Autodesk Inventor part; units mm, degrees
(part 3 of 3)
  spline S74 degree 3 poles (635.3276, -322.5137) (634.4201, -321.4591) (632.6051, -319.35) (629.8185, -316.2423) (626.9841, -313.1784) (624.099, -310.1618) (621.1497, -307.2086) (618.9244, -305.0061) (617.3793, -303.6029) (616.7979, -302.9531) (616.3991, -302.3815) (616.1608, -301.9167) (615.9496, -301.4385) (615.8138, -300.9335) (615.7143, -300.4207) (615.6711, -299.7252) (615.7494, -299.0281) (615.9357, -298.3567) (616.2141, -297.7178) (616.6068, -296.9422) (616.9684, -296.1515) (617.2943, -295.5356) (617.703, -294.9713) (618.1993, -294.4755) (618.77, -294.0756) (619.2329, -293.8336) (619.7124, -293.625) (620.2179, -293.4919) (620.73, -293.3884) (621.4255, -293.3439) (622.296, -293.3933) (624.3564, -293.7264) (627.4658, -294.093) (631.6136, -294.5575) (635.7709, -294.9324) (639.9336, -295.2381) (644.1007, -295.4791) (646.8813, -295.5831) (648.2716, -295.6351) knots 0 0 0 0 0.062506 0.125011 0.187517 0.250023 0.312528 0.375034 0.390661 0.406272 0.414085 0.421898 0.429707 0.43752 0.44533 0.453144 0.468748 0.476562 0.484374 0.5 0.515626 0.523438 0.531252 0.546856 0.55467 0.56248 0.570293 0.578102 0.585915 0.593728 0.609339 0.624966 0.687472 0.749977 0.812483 0.874989 0.937494 1 1 1 1 projected
  arc A78 (648.2716, -295.6351) -> (652.4116, -286.3832) centre (0, 0) ccw projected
  spline S75 degree 3 poles (652.4116, -286.3832) (651.4464, -285.3812) (649.5159, -283.3772) (646.5595, -280.4306) (643.5578, -277.5304) (640.508, -274.6804) (637.3978, -271.8971) (635.0525, -269.8229) (633.4312, -268.5085) (632.8143, -267.8923) (632.3841, -267.3441) (632.12, -266.8933) (631.8824, -266.4277) (631.7185, -265.9312) (631.5904, -265.4247) (631.5083, -264.7327) (631.5473, -264.0323) (631.6957, -263.3515) (631.9378, -262.6981) (632.2864, -261.9016) (632.6031, -261.0919) (632.894, -260.4587) (633.2704, -259.8724) (633.7381, -259.3495) (634.2855, -258.9182) (634.7342, -258.6507) (635.2012, -258.4155) (635.6984, -258.2543) (636.2039, -258.1223) (636.8958, -258.0388) (637.7677, -258.0393) (639.8435, -258.2563) (642.9686, -258.448) (647.1359, -258.6792) (651.3077, -258.8204) (655.481, -258.8923) (659.655, -258.8992) (662.4371, -258.8472) (663.8282, -258.8212) knots 0 0 0 0 0.062506 0.125011 0.187517 0.250023 0.312528 0.375034 0.390661 0.406272 0.414085 0.421898 0.429707 0.43752 0.44533 0.453144 0.468748 0.476562 0.484374 0.5 0.515626 0.523438 0.531252 0.546856 0.55467 0.56248 0.570293 0.578102 0.585915 0.593728 0.609339 0.624966 0.687472 0.749977 0.812483 0.874989 0.937494 1 1 1 1 projected
  arc A79 (663.8282, -258.8212) -> (667.4429, -249.3517) centre (0, 0) ccw projected
  spline S76 degree 3 poles (667.4429, -249.3517) (666.423, -248.4053) (664.3832, -246.5127) (661.2662, -243.7365) (658.1066, -241.0092) (654.9019, -238.3347) (651.6405, -235.7302) (649.1825, -233.7907) (647.4901, -232.5693) (646.8396, -231.9887) (646.3793, -231.4654) (646.0904, -231.0302) (645.8271, -230.5786) (645.6356, -230.0921) (645.4793, -229.5936) (645.3585, -228.9073) (645.3582, -228.2058) (645.4682, -227.5178) (645.6733, -226.8518) (645.9767, -226.037) (646.2475, -225.2109) (646.5024, -224.5623) (646.8453, -223.9558) (647.2829, -223.4075) (647.8053, -222.9463) (648.2383, -222.654) (648.6914, -222.393) (649.1788, -222.2041) (649.676, -222.044) (650.3622, -221.9218) (651.2327, -221.8734) (653.3175, -221.9737) (656.4484, -221.9899) (660.6221, -221.9871) (664.7953, -221.8941) (668.966, -221.7319) (673.1339, -221.5048) (675.9087, -221.2968) (677.2961, -221.1928) knots 0 0 0 0 0.062506 0.125011 0.187517 0.250023 0.312528 0.375034 0.390661 0.406272 0.414085 0.421898 0.429707 0.43752 0.44533 0.453144 0.468748 0.476562 0.484374 0.5 0.515626 0.523438 0.531252 0.546856 0.55467 0.56248 0.570293 0.578102 0.585915 0.593728 0.609339 0.624966 0.687472 0.749977 0.812483 0.874989 0.937494 1 1 1 1 projected
  arc A80 (677.2961, -221.1928) -> (680.3741, -211.5356) centre (0, 0) ccw projected
  spline S77 degree 3 poles (680.3741, -211.5356) (679.3028, -210.6479) (677.1601, -208.8726) (673.8923, -206.2756) (670.5848, -203.7298) (667.2351, -201.2391) (663.8328, -198.8216) (661.27, -197.023) (659.5117, -195.8984) (658.8297, -195.3552) (658.3408, -194.8585) (658.028, -194.4401) (657.7397, -194.0041) (657.5212, -193.529) (657.3372, -193.0401) (657.1782, -192.3616) (657.1385, -191.6613) (657.2098, -190.9681) (657.3772, -190.2917) (657.6344, -189.4612) (657.8585, -188.6212) (658.0766, -187.9593) (658.385, -187.3345) (658.7912, -186.7626) (659.2869, -186.2728) (659.7028, -185.9567) (660.1405, -185.6707) (660.6166, -185.4548) (661.1041, -185.267) (661.7823, -185.1066) (662.6487, -185.0095) (664.7358, -184.9927) (667.8628, -184.8333) (672.0298, -184.5965) (676.1911, -184.2697) (680.3462, -183.8738) (684.4948, -183.4134) (687.2536, -183.0502) (688.6329, -182.8686) knots 0 0 0 0 0.062506 0.125011 0.187517 0.250023 0.312528 0.375034 0.390661 0.406272 0.414085 0.421898 0.429707 0.43752 0.44533 0.453144 0.468748 0.476562 0.484374 0.5 0.515626 0.523438 0.531252 0.546856 0.55467 0.56248 0.570293 0.578102 0.585915 0.593728 0.609339 0.624966 0.687472 0.749977 0.812483 0.874989 0.937494 1 1 1 1 projected
  arc A81 (688.6329, -182.8686) -> (691.1647, -173.0539) centre (0, 0) ccw projected
  spline S78 degree 3 poles (691.1647, -173.0539) (690.0452, -172.2277) (687.8064, -170.5754) (684.3981, -168.1656) (680.953, -165.8093) (677.469, -163.5103) (673.9365, -161.2874) (671.2769, -159.6353) (669.4583, -158.6111) (668.7469, -158.1069) (668.2309, -157.6385) (667.8951, -157.2383) (667.5829, -156.8191) (667.3381, -156.357) (667.127, -155.8792) (666.9301, -155.2107) (666.8512, -154.5137) (666.8835, -153.8177) (667.0128, -153.1329) (667.223, -152.2893) (667.3996, -151.438) (667.5803, -150.765) (667.8532, -150.1239) (668.2267, -149.5301) (668.6941, -149.0132) (669.0916, -148.6743) (669.5126, -148.3642) (669.9759, -148.122) (670.452, -147.9072) (671.1202, -147.709) (671.9798, -147.5634) (674.0627, -147.4297) (677.1758, -147.0952) (681.3229, -146.6251) (685.4594, -146.0655) (689.5858, -145.4372) (693.702, -144.7449) (696.4361, -144.2276) (697.8031, -143.9689) knots 0 0 0 0 0.062506 0.125011 0.187517 0.250023 0.312528 0.375034 0.390661 0.406272 0.414085 0.421898 0.429707 0.43752 0.44533 0.453144 0.468748 0.476562 0.484374 0.5 0.515626 0.523438 0.531252 0.546856 0.55467 0.56248 0.570293 0.578102 0.585915 0.593728 0.609339 0.624966 0.687472 0.749977 0.812483 0.874989 0.937494 1 1 1 1 projected
  arc A82 (697.8031, -143.9689) -> (699.7805, -134.0277) centre (0, 0) ccw projected
  spline S79 degree 3 poles (699.7805, -134.0277) (698.6166, -133.2656) (696.2886, -131.7414) (692.7506, -129.5266) (689.1788, -127.3671) (685.5713, -125.2671) (681.9197, -123.2458) (679.1716, -121.7454) (677.2985, -120.8247) (676.56, -120.3613) (676.0185, -119.9225) (675.6608, -119.5418) (675.3255, -119.1407) (675.0552, -118.6931) (674.8177, -118.2279) (674.5836, -117.5715) (674.4658, -116.88) (674.459, -116.1832) (674.5497, -115.4923) (674.7123, -114.6382) (674.8409, -113.7784) (674.9835, -113.0963) (675.22, -112.4409) (675.5596, -111.8271) (675.9973, -111.2848) (676.3752, -110.9241) (676.7782, -110.5909) (677.2271, -110.3231) (677.6905, -110.0819) (678.3465, -109.8466) (679.1966, -109.6531) (681.2687, -109.4027) (684.3582, -108.8942) (688.4724, -108.1923) (692.571, -107.4016) (696.6556, -106.5431) (700.7266, -105.621) (703.4274, -104.9512) (704.7778, -104.6163) knots 0 0 0 0 0.062506 0.125011 0.187517 0.250023 0.312528 0.375034 0.390661 0.406272 0.414085 0.421898 0.429707 0.43752 0.44533 0.453144 0.468748 0.476562 0.484374 0.5 0.515626 0.523438 0.531252 0.546856 0.55467 0.56248 0.570293 0.578102 0.585915 0.593728 0.609339 0.624966 0.687472 0.749977 0.812483 0.874989 0.937494 1 1 1 1 projected
  arc A83 (704.7778, -104.6163) -> (706.1947, -94.5799) centre (0, 0) ccw projected
  spline S80 degree 3 poles (706.1947, -94.5799) (704.9898, -93.8842) (702.58, -92.4929) (698.9234, -90.48) (695.2361, -88.5241) (691.5166, -86.6297) (687.7574, -84.8163) (684.9295, -83.4724) (683.0077, -82.6582) (682.2443, -82.2369) (681.6791, -81.8292) (681.3006, -81.4691) (680.9434, -81.0875) (680.6484, -80.6558) (680.3852, -80.2045) (680.1147, -79.5623) (679.9583, -78.8785) (679.9124, -78.1832) (679.9642, -77.4883) (680.0787, -76.6265) (680.1588, -75.7608) (680.263, -75.0717) (680.4624, -74.4041) (680.7671, -73.7722) (681.1737, -73.2063) (681.5307, -72.825) (681.9144, -72.4697) (682.3476, -72.1771) (682.7967, -71.9103) (683.4385, -71.6386) (684.2764, -71.3977) (686.3312, -71.0316) (689.3873, -70.3506) (693.4557, -69.4192) (697.5035, -68.3999) (701.5336, -67.3136) (705.5465, -66.1648) (708.2054, -65.3446) (709.5349, -64.9345) knots 0 0 0 0 0.062506 0.125011 0.187517 0.250023 0.312528 0.375034 0.390661 0.406272 0.414085 0.421898 0.429707 0.43752 0.44533 0.453144 0.468748 0.476562 0.484374 0.5 0.515626 0.523438 0.531252 0.546856 0.55467 0.56248 0.570293 0.578102 0.585915 0.593728 0.609339 0.624966 0.687472 0.749977 0.812483 0.874989 0.937494 1 1 1 1 projected
  arc A84 (709.5349, -64.9345) -> (710.3868, -54.8344) centre (0, 0) ccw projected
  spline S81 degree 3 poles (710.3868, -54.8344) (709.1448, -54.2075) (706.6608, -52.9535) (702.8971, -51.1487) (699.1059, -49.4027) (695.286, -47.7198) (691.4311, -46.12) (688.5323, -44.9368) (686.5679, -44.2317) (685.7821, -43.8538) (685.1949, -43.4784) (684.7968, -43.1401) (684.4188, -42.7791) (684.1, -42.3646) (683.8119, -41.9289) (683.5058, -41.3028) (683.3113, -40.6288) (683.2266, -39.9372) (683.2393, -39.2405) (683.3053, -38.3736) (683.3367, -37.5048) (683.4021, -36.811) (683.5638, -36.1332) (683.8325, -35.4853) (684.2068, -34.8974) (684.5419, -34.4967) (684.905, -34.1205) (685.3211, -33.8041) (685.7546, -33.5125) (686.3801, -33.2052) (687.2032, -32.9177) (689.2343, -32.4369) (692.2473, -31.5857) (696.2572, -30.4276) (700.2414, -29.183) (704.2043, -27.8724) (708.1464, -26.5004) (710.7552, -25.5324) (712.0596, -25.0484) knots 0 0 0 0 0.062506 0.125011 0.187517 0.250023 0.312528 0.375034 0.390661 0.406272 0.414085 0.421898 0.429707 0.43752 0.44533 0.453144 0.468748 0.476562 0.484374 0.5 0.515626 0.523438 0.531252 0.546856 0.55467 0.56248 0.570293 0.578102 0.585915 0.593728 0.609339 0.624966 0.687472 0.749977 0.812483 0.874989 0.937494 1 1 1 1 projected
  arc A85 (712.0596, -25.0484) -> (712.3438, -14.9165) centre (0, 0) ccw projected
  spline S82 degree 3 poles (712.3438, -14.9165) (711.0686, -14.3601) (708.5182, -13.2474) (704.6592, -11.6564) (700.7761, -10.1258) (696.8679, -8.6597) (692.9293, -7.2786) (689.9687, -6.2598) (687.9678, -5.6659) (687.1621, -5.3327) (686.5548, -4.9908) (686.1384, -4.6754) (685.7407, -4.3362) (685.3992, -3.9402) (685.0871, -3.5213) (684.7464, -2.9134) (684.5144, -2.2513) (684.391, -1.5656) (684.3646, -0.8692) (684.3819, 0) (684.3646, 0.8692) (684.391, 1.5656) (684.5144, 2.2513) (684.7464, 2.9134) (685.0871, 3.5213) (685.3992, 3.9402) (685.7407, 4.3362) (686.1384, 4.6754) (686.5548, 4.9908) (687.1621, 5.3327) (687.9678, 5.6659) (689.9687, 6.2598) (692.9293, 7.2786) (696.8679, 8.6597) (700.7761, 10.1258) (704.6592, 11.6564) (708.5182, 13.2474) (711.0686, 14.3601) (712.3438, 14.9165) knots 0 0 0 0 0.062506 0.125011 0.187517 0.250023 0.312528 0.375034 0.390661 0.406272 0.414085 0.421898 0.429707 0.43752 0.44533 0.453144 0.468748 0.476562 0.484374 0.5 0.515626 0.523438 0.531252 0.546856 0.55467 0.56248 0.570293 0.578102 0.585915 0.593728 0.609339 0.624966 0.687472 0.749977 0.812483 0.874989 0.937494 1 1 1 1 projected
  arc A86 (712.3438, 14.9165) -> (712.0596, 25.0484) centre (0, 0) ccw projected
  spline S83 degree 3 poles (712.0596, 25.0484) (710.7552, 25.5324) (708.1464, 26.5004) (704.2043, 27.8724) (700.2414, 29.183) (696.2572, 30.4276) (692.2473, 31.5857) (689.2343, 32.4369) (687.2032, 32.9177) (686.3801, 33.2052) (685.7546, 33.5125) (685.3211, 33.8041) (684.905, 34.1205) (684.5419, 34.4967) (684.2068, 34.8974) (683.8325, 35.4853) (683.5638, 36.1332) (683.4021, 36.811) (683.3367, 37.5048) (683.3053, 38.3736) (683.2393, 39.2405) (683.2266, 39.9372) (683.3113, 40.6288) (683.5058, 41.3028) (683.8119, 41.9289) (684.1, 42.3646) (684.4188, 42.7791) (684.7968, 43.1401) (685.1949, 43.4784) (685.7821, 43.8538) (686.5679, 44.2317) (688.5323, 44.9368) (691.4311, 46.12) (695.286, 47.7198) (699.1059, 49.4027) (702.8971, 51.1487) (706.6608, 52.9535) (709.1448, 54.2075) (710.3868, 54.8344) knots 0 0 0 0 0.062506 0.125011 0.187517 0.250023 0.312528 0.375034 0.390661 0.406272 0.414085 0.421898 0.429707 0.43752 0.44533 0.453144 0.468748 0.476562 0.484374 0.5 0.515626 0.523438 0.531252 0.546856 0.55467 0.56248 0.570293 0.578102 0.585915 0.593728 0.609339 0.624966 0.687472 0.749977 0.812483 0.874989 0.937494 1 1 1 1 projected
  arc A87 (710.3868, 54.8344) -> (709.5349, 64.9345) centre (0, 0) ccw projected
  spline S84 degree 3 poles (709.5349, 64.9345) (708.2054, 65.3446) (705.5465, 66.1648) (701.5336, 67.3136) (697.5035, 68.3999) (693.4557, 69.4192) (689.3873, 70.3506) (686.3312, 71.0316) (684.2764, 71.3977) (683.4385, 71.6386) (682.7967, 71.9103) (682.3476, 72.1771) (681.9144, 72.4697) (681.5307, 72.825) (681.1737, 73.2063) (680.7671, 73.7722) (680.4624, 74.4041) (680.263, 75.0717) (680.1588, 75.7608) (680.0787, 76.6265) (679.9642, 77.4883) (679.9124, 78.1832) (679.9583, 78.8785) (680.1147, 79.5623) (680.3852, 80.2045) (680.6484, 80.6558) (680.9434, 81.0875) (681.3006, 81.4691) (681.6791, 81.8292) (682.2443, 82.2369) (683.0077, 82.6582) (684.9295, 83.4724) (687.7574, 84.8163) (691.5166, 86.6297) (695.2361, 88.5241) (698.9234, 90.48) (702.58, 92.4929) (704.9898, 93.8842) (706.1947, 94.5799) knots 0 0 0 0 0.062506 0.125011 0.187517 0.250023 0.312528 0.375034 0.390661 0.406272 0.414085 0.421898 0.429707 0.43752 0.44533 0.453144 0.468748 0.476562 0.484374 0.5 0.515626 0.523438 0.531252 0.546856 0.55467 0.56248 0.570293 0.578102 0.585915 0.593728 0.609339 0.624966 0.687472 0.749977 0.812483 0.874989 0.937494 1 1 1 1 projected
  arc A88 (706.1947, 94.5799) -> (704.7778, 104.6163) centre (0, 0) ccw projected
  spline S85 degree 3 poles (704.7778, 104.6163) (703.4274, 104.9512) (700.7266, 105.621) (696.6556, 106.5431) (692.571, 107.4016) (688.4724, 108.1923) (684.3582, 108.8942) (681.2687, 109.4027) (679.1966, 109.6531) (678.3465, 109.8466) (677.6905, 110.0819) (677.2271, 110.3231) (676.7782, 110.5909) (676.3752, 110.9241) (675.9973, 111.2848) (675.5596, 111.8271) (675.22, 112.4409) (674.9835, 113.0963) (674.8409, 113.7784) (674.7123, 114.6382) (674.5497, 115.4923) (674.459, 116.1832) (674.4658, 116.88) (674.5836, 117.5715) (674.8177, 118.2279) (675.0552, 118.6931) (675.3255, 119.1407) (675.6608, 119.5418) (676.0185, 119.9225) (676.56, 120.3613) (677.2985, 120.8247) (679.1716, 121.7454) (681.9197, 123.2458) (685.5713, 125.2671) (689.1788, 127.3671) (692.7506, 129.5266) (696.2886, 131.7414) (698.6166, 133.2656) (699.7805, 134.0277) knots 0 0 0 0 0.062506 0.125011 0.187517 0.250023 0.312528 0.375034 0.390661 0.406272 0.414085 0.421898 0.429707 0.43752 0.44533 0.453144 0.468748 0.476562 0.484374 0.5 0.515626 0.523438 0.531252 0.546856 0.55467 0.56248 0.570293 0.578102 0.585915 0.593728 0.609339 0.624966 0.687472 0.749977 0.812483 0.874989 0.937494 1 1 1 1 projected
  arc A89 (699.7805, 134.0277) -> (697.8031, 143.9689) centre (0, 0) ccw projected
  spline S86 degree 3 poles (697.8031, 143.9689) (696.4361, 144.2276) (693.702, 144.7449) (689.5858, 145.4372) (685.4594, 146.0655) (681.3229, 146.6251) (677.1758, 147.0952) (674.0627, 147.4297) (671.9798, 147.5634) (671.1202, 147.709) (670.452, 147.9072) (669.9759, 148.122) (669.5126, 148.3642) (669.0916, 148.6743) (668.6941, 149.0132) (668.2267, 149.5301) (667.8532, 150.1239) (667.5803, 150.765) (667.3996, 151.438) (667.223, 152.2893) (667.0128, 153.1329) (666.8835, 153.8177) (666.8512, 154.5137) (666.9301, 155.2107) (667.127, 155.8792) (667.3381, 156.357) (667.5829, 156.8191) (667.8951, 157.2383) (668.2309, 157.6385) (668.7469, 158.1069) (669.4583, 158.6111) (671.2769, 159.6353) (673.9365, 161.2874) (677.469, 163.5103) (680.953, 165.8093) (684.3981, 168.1656) (687.8064, 170.5754) (690.0452, 172.2277) (691.1647, 173.0539) knots 0 0 0 0 0.062506 0.125011 0.187517 0.250023 0.312528 0.375034 0.390661 0.406272 0.414085 0.421898 0.429707 0.43752 0.44533 0.453144 0.468748 0.476562 0.484374 0.5 0.515626 0.523438 0.531252 0.546856 0.55467 0.56248 0.570293 0.578102 0.585915 0.593728 0.609339 0.624966 0.687472 0.749977 0.812483 0.874989 0.937494 1 1 1 1 projected
  arc A90 (691.1647, 173.0539) -> (688.6329, 182.8686) centre (0, 0) ccw projected
  spline S87 degree 3 poles (688.6329, 182.8686) (687.2536, 183.0502) (684.4948, 183.4134) (680.3462, 183.8738) (676.1911, 184.2697) (672.0298, 184.5965) (667.8628, 184.8333) (664.7358, 184.9927) (662.6487, 185.0095) (661.7823, 185.1066) (661.1041, 185.267) (660.6166, 185.4548) (660.1405, 185.6707) (659.7028, 185.9567) (659.2869, 186.2728) (658.7912, 186.7626) (658.385, 187.3345) (658.0766, 187.9593) (657.8585, 188.6212) (657.6344, 189.4612) (657.3772, 190.2917) (657.2098, 190.9681) (657.1385, 191.6613) (657.1782, 192.3616) (657.3372, 193.0401) (657.5212, 193.529) (657.7397, 194.0041) (658.028, 194.4401) (658.3408, 194.8585) (658.8297, 195.3552) (659.5117, 195.8984) (661.27, 197.023) (663.8328, 198.8216) (667.2351, 201.2391) (670.5848, 203.7298) (673.8923, 206.2756) (677.1601, 208.8726) (679.3028, 210.6479) (680.3741, 211.5356) knots 0 0 0 0 0.062506 0.125011 0.187517 0.250023 0.312528 0.375034 0.390661 0.406272 0.414085 0.421898 0.429707 0.43752 0.44533 0.453144 0.468748 0.476562 0.484374 0.5 0.515626 0.523438 0.531252 0.546856 0.55467 0.56248 0.570293 0.578102 0.585915 0.593728 0.609339 0.624966 0.687472 0.749977 0.812483 0.874989 0.937494 1 1 1 1 projected
  arc A91 (680.3741, 211.5356) -> (677.2961, 221.1928) centre (0, 0) ccw projected
  spline S88 degree 3 poles (677.2961, 221.1928) (675.9087, 221.2968) (673.1339, 221.5048) (668.966, 221.7319) (664.7953, 221.8941) (660.6221, 221.9871) (656.4484, 221.9899) (653.3175, 221.9737) (651.2327, 221.8734) (650.3622, 221.9218) (649.676, 222.044) (649.1788, 222.2041) (648.6914, 222.393) (648.2383, 222.654) (647.8053, 222.9463) (647.2829, 223.4075) (646.8453, 223.9558) (646.5024, 224.5623) (646.2475, 225.2109) (645.9767, 226.037) (645.6733, 226.8518) (645.4682, 227.5178) (645.3582, 228.2058) (645.3585, 228.9073) (645.4793, 229.5936) (645.6356, 230.0921) (645.8271, 230.5786) (646.0904, 231.0302) (646.3793, 231.4654) (646.8396, 231.9887) (647.4901, 232.5693) (649.1825, 233.7907) (651.6405, 235.7302) (654.9019, 238.3347) (658.1066, 241.0092) (661.2662, 243.7365) (664.3832, 246.5127) (666.423, 248.4053) (667.4429, 249.3517) knots 0 0 0 0 0.062506 0.125011 0.187517 0.250023 0.312528 0.375034 0.390661 0.406272 0.414085 0.421898 0.429707 0.43752 0.44533 0.453144 0.468748 0.476562 0.484374 0.5 0.515626 0.523438 0.531252 0.546856 0.55467 0.56248 0.570293 0.578102 0.585915 0.593728 0.609339 0.624966 0.687472 0.749977 0.812483 0.874989 0.937494 1 1 1 1 projected
  arc A92 (667.4429, 249.3517) -> (663.8282, 258.8212) centre (0, 0) ccw projected
  spline S89 degree 3 poles (663.8282, 258.8212) (662.4371, 258.8472) (659.655, 258.8992) (655.481, 258.8923) (651.3077, 258.8204) (647.1359, 258.6792) (642.9686, 258.448) (639.8435, 258.2563) (637.7677, 258.0393) (636.8958, 258.0388) (636.2039, 258.1223) (635.6984, 258.2543) (635.2012, 258.4155) (634.7342, 258.6507) (634.2855, 258.9182) (633.7381, 259.3495) (633.2704, 259.8724) (632.894, 260.4587) (632.6031, 261.0919) (632.2864, 261.9016) (631.9378, 262.6981) (631.6957, 263.3515) (631.5473, 264.0323) (631.5083, 264.7327) (631.5904, 265.4247) (631.7185, 265.9312) (631.8824, 266.4277) (632.12, 266.8933) (632.3841, 267.3441) (632.8143, 267.8923) (633.4312, 268.5085) (635.0525, 269.8229) (637.3978, 271.8971) (640.508, 274.6804) (643.5578, 277.5304) (646.5595, 280.4306) (649.5159, 283.3772) (651.4464, 285.3812) (652.4116, 286.3832) knots 0 0 0 0 0.062506 0.125011 0.187517 0.250023 0.312528 0.375034 0.390661 0.406272 0.414085 0.421898 0.429707 0.43752 0.44533 0.453144 0.468748 0.476562 0.484374 0.5 0.515626 0.523438 0.531252 0.546856 0.55467 0.56248 0.570293 0.578102 0.585915 0.593728 0.609339 0.624966 0.687472 0.749977 0.812483 0.874989 0.937494 1 1 1 1 projected
  arc A93 (652.4116, 286.3832) -> (648.2716, 295.6351) centre (0, 0) ccw projected
  spline S90 degree 3 poles (648.2716, 295.6351) (646.8813, 295.5831) (644.1007, 295.4791) (639.9336, 295.2381) (635.7709, 294.9324) (631.6136, 294.5575) (627.4658, 294.093) (624.3564, 293.7264) (622.296, 293.3933) (621.4255, 293.3439) (620.73, 293.3884) (620.2179, 293.4919) (619.7124, 293.625) (619.2329, 293.8336) (618.77, 294.0756) (618.1993, 294.4755) (617.703, 294.9713) (617.2943, 295.5356) (616.9684, 296.1515) (616.6068, 296.9422) (616.2141, 297.7178) (615.9357, 298.3567) (615.7494, 299.0281) (615.6711, 299.7252) (615.7143, 300.4207) (615.8138, 300.9335) (615.9496, 301.4385) (616.1608, 301.9167) (616.3991, 302.3815) (616.7979, 302.9531) (617.3793, 303.6029) (618.9244, 305.0061) (621.1497, 307.2086) (624.099, 310.1618) (626.9841, 313.1784) (629.8185, 316.2423) (632.6051, 319.35) (634.4201, 321.4591) (635.3276, 322.5137) knots 0 0 0 0 0.062506 0.125011 0.187517 0.250023 0.312528 0.375034 0.390661 0.406272 0.414085 0.421898 0.429707 0.43752 0.44533 0.453144 0.468748 0.476562 0.484374 0.5 0.515626 0.523438 0.531252 0.546856 0.55467 0.56248 0.570293 0.578102 0.585915 0.593728 0.609339 0.624966 0.687472 0.749977 0.812483 0.874989 0.937494 1 1 1 1 projected
  arc A94 (635.3276, 322.5137) -> (630.6754, 331.5189) centre (0, 0) ccw projected
  spline S91 degree 3 poles (630.6754, 331.5189) (629.2902, 331.389) (626.5198, 331.1292) (622.3727, 330.655) (618.2337, 330.1163) (614.104, 329.509) (609.9888, 328.8126) (606.9048, 328.2722) (604.8663, 327.8241) (603.9999, 327.726) (603.303, 327.7315) (602.786, 327.8061) (602.2738, 327.9106) (601.7834, 328.092) (601.3076, 328.3077) (600.7153, 328.6749) (600.1921, 329.1421) (599.7524, 329.6826) (599.3924, 330.2793) (598.9871, 331.0485) (598.5515, 331.8009) (598.2378, 332.4231) (598.014, 333.083) (597.8968, 333.7746) (597.901, 334.4715) (597.9715, 334.9891) (598.0788, 335.5008) (598.2628, 335.9901) (598.4747, 336.4676) (598.8409, 337.0606) (599.3849, 337.742) (600.8488, 339.2296) (602.9472, 341.5534) (605.7262, 344.6674) (608.4377, 347.841) (611.0958, 351.059) (613.7038, 354.3181) (615.3977, 356.5256) (616.2446, 357.6294) knots 0 0 0 0 0.062506 0.125011 0.187517 0.250023 0.312528 0.375034 0.390661 0.406272 0.414085 0.421898 0.429707 0.43752 0.44533 0.453144 0.468748 0.476562 0.484374 0.5 0.515626 0.523438 0.531252 0.546856 0.55467 0.56248 0.570293 0.578102 0.585915 0.593728 0.609339 0.624966 0.687472 0.749977 0.812483 0.874989 0.937494 1 1 1 1 projected
  arc A95 (616.2446, 357.6294) -> (611.0948, 366.3596) centre (0, 0) ccw projected
  spline S92 degree 3 poles (611.0948, 366.3596) (609.7191, 366.1523) (606.9676, 365.7376) (602.8536, 365.0315) (598.7514, 364.2616) (594.6622, 363.4237) (590.5925, 362.4976) (587.5436, 361.7852) (585.5335, 361.2235) (584.674, 361.077) (583.9779, 361.0434) (583.4575, 361.0889) (582.9402, 361.1645) (582.4404, 361.3181) (581.9532, 361.5068) (581.3414, 361.8402) (580.7927, 362.2774) (580.3234, 362.7924) (579.9306, 363.3679) (579.4827, 364.1131) (579.0056, 364.8399) (578.6575, 365.4436) (578.3971, 366.0899) (578.2414, 366.7739) (578.2064, 367.4699) (578.2478, 367.9906) (578.3263, 368.5076) (578.4825, 369.0064) (578.6673, 369.495) (578.9997, 370.1076) (579.5046, 370.8184) (580.8828, 372.3858) (582.8476, 374.8236) (585.4477, 378.0885) (587.9769, 381.4091) (590.4504, 384.7711) (592.8715, 388.1713) (594.439, 390.4704) (595.2227, 391.6199) knots 0 0 0 0 0.062506 0.125011 0.187517 0.250023 0.312528 0.375034 0.390661 0.406272 0.414085 0.421898 0.429707 0.43752 0.44533 0.453144 0.468748 0.476562 0.484374 0.5 0.515626 0.523438 0.531252 0.546856 0.55467 0.56248 0.570293 0.578102 0.585915 0.593728 0.609339 0.624966 0.687472 0.749977 0.812483 0.874989 0.937494 1 1 1 1 projected
  arc A96 (595.2227, 391.6199) -> (589.5915, 400.0476) centre (0, 0) ccw projected
  spline S93 degree 3 poles (589.5915, 400.0476) (588.2295, 399.7635) (585.5056, 399.1951) (581.4377, 398.2595) (577.3851, 397.2608) (573.3493, 396.1949) (569.338, 395.0422) (566.3339, 394.1599) (564.3583, 393.4864) (563.5084, 393.2919) (562.8153, 393.2193) (562.2931, 393.2355) (561.7725, 393.2821) (561.2648, 393.4074) (560.7679, 393.5684) (560.1383, 393.8671) (559.566, 394.2727) (559.0685, 394.7606) (558.644, 395.3133) (558.1551, 396.0322) (557.638, 396.7311) (557.2566, 397.3143) (556.9604, 397.945) (556.7665, 398.6191) (556.6926, 399.312) (556.7047, 399.8343) (556.7541, 400.3549) (556.8821, 400.8617) (557.0392, 401.3599) (557.3367, 401.9901) (557.801, 402.7281) (559.0892, 404.3703) (560.9141, 406.9145) (563.327, 410.32) (565.6661, 413.7772) (567.9472, 417.2726) (570.1739, 420.8032) (571.61, 423.1866) (572.328, 424.3782) knots 0 0 0 0 0.062506 0.125011 0.187517 0.250023 0.312528 0.375034 0.390661 0.406272 0.414085 0.421898 0.429707 0.43752 0.44533 0.453144 0.468748 0.476562 0.484374 0.5 0.515626 0.523438 0.531252 0.546856 0.55467 0.56248 0.570293 0.578102 0.585915 0.593728 0.609339 0.624966 0.687472 0.749977 0.812483 0.874989 0.937494 1 1 1 1 projected
  arc A97 (572.328, 424.3782) -> (566.2331, 432.4769) centre (0, 0) ccw projected
  spline S94 degree 3 poles (566.2331, 432.4769) (564.8892, 432.1169) (562.2015, 431.3967) (558.1924, 430.2345) (554.2022, 429.0101) (550.2325, 427.7196) (546.2921, 426.3437) (543.3422, 425.2944) (541.4076, 424.5112) (540.5699, 424.2693) (539.8819, 424.158) (539.3597, 424.1449) (538.8372, 424.1622) (538.3233, 424.2589) (537.8181, 424.3918) (537.1728, 424.6546) (536.5786, 425.0276) (536.0546, 425.4868) (535.5998, 426.0148) (535.0713, 426.7051) (534.5159, 427.374) (534.1023, 427.9349) (533.7712, 428.5479) (533.5398, 429.2102) (533.4272, 429.8979) (533.41, 430.42) (533.4301, 430.9425) (533.5296, 431.4557) (533.6585, 431.9619) (533.9201, 432.6078) (534.3423, 433.3707) (535.5364, 435.0826) (537.2158, 437.725) (539.434, 441.2605) (541.5755, 444.8434) (543.6571, 448.4612) (545.6823, 452.1111) (546.9825, 454.5712) (547.6326, 455.8013) knots 0 0 0 0 0.062506 0.125011 0.187517 0.250023 0.312528 0.375034 0.390661 0.406272 0.414085 0.421898 0.429707 0.43752 0.44533 0.453144 0.468748 0.476562 0.484374 0.5 0.515626 0.523438 0.531252 0.546856 0.55467 0.56248 0.570293 0.578102 0.585915 0.593728 0.609339 0.624966 0.687472 0.749977 0.812483 0.874989 0.937494 1 1 1 1 projected
  arc A98 (547.6326, 455.8013) -> (541.0931, 463.5455) centre (0, 0) ccw projected
  spline S95 degree 3 poles (541.0931, 463.5455) (539.7716, 463.1107) (537.1284, 462.2409) (533.1909, 460.8557) (529.2755, 459.4096) (525.3845, 457.8985) (521.5274, 456.3038) (518.641, 455.0908) (516.7533, 454.2003) (515.9305, 453.9119) (515.2498, 453.7621) (514.7292, 453.7198) (514.2066, 453.7077) (513.6881, 453.7755) (513.1762, 453.8798) (512.5171, 454.1061) (511.903, 454.4451) (511.354, 454.8742) (510.8703, 455.3759) (510.304, 456.0355) (509.7119, 456.6722) (509.2676, 457.209) (508.9026, 457.8025) (508.6345, 458.4508) (508.4834, 459.131) (508.4371, 459.6514) (508.4278, 460.1742) (508.4983, 460.6921) (508.5986, 461.2048) (508.8237, 461.8644) (509.2024, 462.6498) (510.2986, 464.4259) (511.8272, 467.1583) (513.8437, 470.8126) (515.781, 474.51) (517.6564, 478.2388) (519.4737, 481.9965) (520.634, 484.5257) (521.2141, 485.7902) knots 0 0 0 0 0.062506 0.125011 0.187517 0.250023 0.312528 0.375034 0.390661 0.406272 0.414085 0.421898 0.429707 0.43752 0.44533 0.453144 0.468748 0.476562 0.484374 0.5 0.515626 0.523438 0.531252 0.546856 0.55467 0.56248 0.570293 0.578102 0.585915 0.593728 0.609339 0.624966 0.687472 0.749977 0.812483 0.874989 0.937494 1 1 1 1 projected
  arc A99 (521.2141, 485.7902) -> (514.2507, 493.1556) centre (0, 0) ccw projected
  spline S96 degree 3 poles (514.2507, 493.1556) (512.9556, 492.6473) (510.3654, 491.6307) (506.5117, 490.027) (502.6836, 488.3636) (498.8834, 486.6367) (495.1218, 484.8283) (492.3079, 483.4553) (490.4731, 482.4603) (489.6678, 482.1262) (488.9966, 481.9385) (488.4791, 481.8671) (487.958, 481.8258) (487.4366, 481.8643) (486.9196, 481.9398) (486.2489, 482.1288) (485.6167, 482.4328) (485.0446, 482.8305) (484.5335, 483.3042) (483.9311, 483.9311) (483.3042, 484.5335) (482.8305, 485.0446) (482.4328, 485.6167) (482.1288, 486.2489) (481.9398, 486.9196) (481.8643, 487.4366) (481.8258, 487.958) (481.8671, 488.4791) (481.9385, 488.9966) (482.1262, 489.6678) (482.4603, 490.4731) (483.4553, 492.3079) (484.8283, 495.1218) (486.6367, 498.8834) (488.3636, 502.6836) (490.027, 506.5117) (491.6307, 510.3654) (492.6473, 512.9556) (493.1556, 514.2507) knots 0 0 0 0 0.062506 0.125011 0.187517 0.250023 0.312528 0.375034 0.390661 0.406272 0.414085 0.421898 0.429707 0.43752 0.44533 0.453144 0.468748 0.476562 0.484374 0.5 0.515626 0.523438 0.531252 0.546856 0.55467 0.56248 0.570293 0.578102 0.585915 0.593728 0.609339 0.624966 0.687472 0.749977 0.812483 0.874989 0.937494 1 1 1 1 projected
  arc A100 (493.1556, 514.2507) -> (485.7902, 521.2141) centre (0, 0) ccw projected
  spline S97 degree 3 poles (485.7902, 521.2141) (484.5257, 520.634) (481.9965, 519.4737) (478.2388, 517.6564) (474.51, 515.781) (470.8126, 513.8437) (467.1583, 511.8272) (464.4259, 510.2986) (462.6498, 509.2024) (461.8644, 508.8237) (461.2048, 508.5986) (460.6921, 508.4983) (460.1742, 508.4278) (459.6514, 508.4371) (459.131, 508.4834) (458.4508, 508.6345) (457.8025, 508.9026) (457.209, 509.2676) (456.6722, 509.7119) (456.0355, 510.304) (455.3759, 510.8703) (454.8742, 511.354) (454.4451, 511.903) (454.1061, 512.5171) (453.8798, 513.1762) (453.7755, 513.6881) (453.7077, 514.2066) (453.7198, 514.7292) (453.7621, 515.2498) (453.9119, 515.9305) (454.2003, 516.7533) (455.0908, 518.641) (456.3038, 521.5274) (457.8985, 525.3845) (459.4096, 529.2755) (460.8557, 533.1909) (462.2409, 537.1284) (463.1107, 539.7716) (463.5455, 541.0931) knots 0 0 0 0 0.062506 0.125011 0.187517 0.250023 0.312528 0.375034 0.390661 0.406272 0.414085 0.421898 0.429707 0.43752 0.44533 0.453144 0.468748 0.476562 0.484374 0.5 0.515626 0.523438 0.531252 0.546856 0.55467 0.56248 0.570293 0.578102 0.585915 0.593728 0.609339 0.624966 0.687472 0.749977 0.812483 0.874989 0.937494 1 1 1 1 projected
  arc A101 (463.5455, 541.0931) -> (455.8013, 547.6326) centre (0, 0) ccw projected
  spline S98 degree 3 poles (455.8013, 547.6326) (454.5712, 546.9825) (452.1111, 545.6823) (448.4612, 543.6571) (444.8434, 541.5755) (441.2605, 539.434) (437.725, 537.2158) (435.0826, 535.5364) (433.3707, 534.3423) (432.6078, 533.9201) (431.9619, 533.6585) (431.4557, 533.5296) (430.9425, 533.4301) (430.42, 533.41) (429.8979, 533.4272) (429.2102, 533.5398) (428.5479, 533.7712) (427.9349, 534.1023) (427.374, 534.5159) (426.7051, 535.0713) (426.0148, 535.5998) (425.4868, 536.0546) (425.0276, 536.5786) (424.6546, 537.1728) (424.3918, 537.8181) (424.2589, 538.3233) (424.1622, 538.8372) (424.1449, 539.3597) (424.158, 539.8819) (424.2693, 540.5699) (424.5112, 541.4076) (425.2944, 543.3422) (426.3437, 546.2921) (427.7196, 550.2325) (429.0101, 554.2022) (430.2345, 558.1924) (431.3967, 562.2015) (432.1169, 564.8892) (432.4769, 566.2331) knots 0 0 0 0 0.062506 0.125011 0.187517 0.250023 0.312528 0.375034 0.390661 0.406272 0.414085 0.421898 0.429707 0.43752 0.44533 0.453144 0.468748 0.476562 0.484374 0.5 0.515626 0.523438 0.531252 0.546856 0.55467 0.56248 0.570293 0.578102 0.585915 0.593728 0.609339 0.624966 0.687472 0.749977 0.812483 0.874989 0.937494 1 1 1 1 projected
  arc A102 (432.4769, 566.2331) -> (424.3782, 572.328) centre (0, 0) ccw projected
  spline S99 degree 3 poles (424.3782, 572.328) (423.1866, 571.61) (420.8032, 570.1739) (417.2726, 567.9472) (413.7772, 565.6661) (410.32, 563.327) (406.9145, 560.9141) (404.3703, 559.0892) (402.7281, 557.801) (401.9901, 557.3367) (401.3599, 557.0392) (400.8617, 556.8821) (400.3549, 556.7541) (399.8343, 556.7047) (399.312, 556.6926) (398.6191, 556.7665) (397.945, 556.9604) (397.3143, 557.2566) (396.7311, 557.638) (396.0322, 558.1551) (395.3133, 558.644) (394.7606, 559.0685) (394.2727, 559.566) (393.8671, 560.1383) (393.5684, 560.7679) (393.4074, 561.2648) (393.2821, 561.7725) (393.2355, 562.2931) (393.2193, 562.8153) (393.2919, 563.5084) (393.4864, 564.3583) (394.1599, 566.3339) (395.0422, 569.338) (396.1949, 573.3493) (397.2608, 577.3851) (398.2595, 581.4377) (399.1951, 585.5056) (399.7635, 588.2295) (400.0476, 589.5915) knots 0 0 0 0 0.062506 0.125011 0.187517 0.250023 0.312528 0.375034 0.390661 0.406272 0.414085 0.421898 0.429707 0.43752 0.44533 0.453144 0.468748 0.476562 0.484374 0.5 0.515626 0.523438 0.531252 0.546856 0.55467 0.56248 0.570293 0.578102 0.585915 0.593728 0.609339 0.624966 0.687472 0.749977 0.812483 0.874989 0.937494 1 1 1 1 projected
  arc A103 (400.0476, 589.5915) -> (391.6199, 595.2227) centre (0, 0) ccw projected
  spline S100 degree 3 poles (391.6199, 595.2227) (390.4704, 594.439) (388.1713, 592.8715) (384.7711, 590.4504) (381.4091, 587.9769) (378.0885, 585.4477) (374.8236, 582.8476) (372.3858, 580.8828) (370.8184, 579.5046) (370.1076, 578.9997) (369.495, 578.6673) (369.0064, 578.4825) (368.5076, 578.3263) (367.9906, 578.2478) (367.4699, 578.2064) (366.7739, 578.2414) (366.0899, 578.3971) (365.4436, 578.6575) (364.8399, 579.0056) (364.1131, 579.4827) (363.3679, 579.9306) (362.7924, 580.3234) (362.2774, 580.7927) (361.8402, 581.3414) (361.5068, 581.9532) (361.3181, 582.4404) (361.1645, 582.9402) (361.0889, 583.4575) (361.0434, 583.9779) (361.077, 584.674) (361.2235, 585.5335) (361.7852, 587.5436) (362.4976, 590.5925) (363.4237, 594.6622) (364.2616, 598.7514) (365.0315, 602.8536) (365.7376, 606.9676) (366.1523, 609.7191) (366.3596, 611.0948) knots 0 0 0 0 0.062506 0.125011 0.187517 0.250023 0.312528 0.375034 0.390661 0.406272 0.414085 0.421898 0.429707 0.43752 0.44533 0.453144 0.468748 0.476562 0.484374 0.5 0.515626 0.523438 0.531252 0.546856 0.55467 0.56248 0.570293 0.578102 0.585915 0.593728 0.609339 0.624966 0.687472 0.749977 0.812483 0.874989 0.937494 1 1 1 1 projected
  arc A104 (366.3596, 611.0948) -> (357.6294, 616.2446) centre (0, 0) ccw projected
  spline S101 degree 3 poles (357.6294, 616.2446) (356.5256, 615.3977) (354.3181, 613.7038) (351.059, 611.0958) (347.841, 608.4377) (344.6674, 605.7262) (341.5534, 602.9472) (339.2296, 600.8488) (337.742, 599.3849) (337.0606, 598.8409) (336.4676, 598.4747) (335.9901, 598.2628) (335.5008, 598.0788) (334.9891, 597.9715) (334.4715, 597.901) (333.7746, 597.8968) (333.083, 598.014) (332.4231, 598.2378) (331.8009, 598.5515) (331.0485, 598.9871) (330.2793, 599.3924) (329.6826, 599.7524) (329.1421, 600.1921) (328.6749, 600.7153) (328.3077, 601.3076) (328.092, 601.7834) (327.9106, 602.2738) (327.8061, 602.786) (327.7315, 603.303) (327.726, 603.9999) (327.8241, 604.8663) (328.2722, 606.9048) (328.8126, 609.9888) (329.509, 614.104) (330.1163, 618.2337) (330.655, 622.3727) (331.1292, 626.5198) (331.389, 629.2902) (331.5189, 630.6754) knots 0 0 0 0 0.062506 0.125011 0.187517 0.250023 0.312528 0.375034 0.390661 0.406272 0.414085 0.421898 0.429707 0.43752 0.44533 0.453144 0.468748 0.476562 0.484374 0.5 0.515626 0.523438 0.531252 0.546856 0.55467 0.56248 0.570293 0.578102 0.585915 0.593728 0.609339 0.624966 0.687472 0.749977 0.812483 0.874989 0.937494 1 1 1 1 projected
  arc A105 (331.5189, 630.6754) -> (322.5137, 635.3276) centre (0, 0) ccw projected
  spline S102 degree 3 poles (322.5137, 635.3276) (321.4591, 634.4201) (319.35, 632.6051) (316.2423, 629.8185) (313.1784, 626.9841) (310.1618, 624.099) (307.2086, 621.1497) (305.0061, 618.9244) (303.6029, 617.3793) (302.9531, 616.7979) (302.3815, 616.3991) (301.9167, 616.1608) (301.4385, 615.9496) (300.9335, 615.8138) (300.4207, 615.7143) (299.7252, 615.6711) (299.0281, 615.7494) (298.3567, 615.9357) (297.7178, 616.2141) (296.9422, 616.6068) (296.1515, 616.9684) (295.5356, 617.2943) (294.9713, 617.703) (294.4755, 618.1993) (294.0756, 618.77) (293.8336, 619.2329) (293.625, 619.7124) (293.4919, 620.2179) (293.3884, 620.73) (293.3439, 621.4255) (293.3933, 622.296) (293.7264, 624.3564) (294.093, 627.4658) (294.5575, 631.6136) (294.9324, 635.7709) (295.2381, 639.9336) (295.4791, 644.1007) (295.5831, 646.8813) (295.6351, 648.2716) knots 0 0 0 0 0.062506 0.125011 0.187517 0.250023 0.312528 0.375034 0.390661 0.406272 0.414085 0.421898 0.429707 0.43752 0.44533 0.453144 0.468748 0.476562 0.484374 0.5 0.515626 0.523438 0.531252 0.546856 0.55467 0.56248 0.570293 0.578102 0.585915 0.593728 0.609339 0.624966 0.687472 0.749977 0.812483 0.874989 0.937494 1 1 1 1 projected
  arc A106 (295.6351, 648.2716) -> (286.3832, 652.4116) centre (0, 0) ccw projected
  spline S103 degree 3 poles (286.3832, 652.4116) (285.3812, 651.4464) (283.3772, 649.5159) (280.4306, 646.5595) (277.5304, 643.5578) (274.6804, 640.508) (271.8971, 637.3978) (269.8229, 635.0525) (268.5085, 633.4312) (267.8923, 632.8143) (267.3441, 632.3841) (266.8933, 632.12) (266.4277, 631.8824) (265.9312, 631.7185) (265.4247, 631.5904) (264.7327, 631.5083) (264.0323, 631.5473) (263.3515, 631.6957) (262.6981, 631.9378) (261.9016, 632.2864) (261.0919, 632.6031) (260.4587, 632.894) (259.8724, 633.2704) (259.3495, 633.7381) (258.9182, 634.2855) (258.6507, 634.7342) (258.4155, 635.2012) (258.2543, 635.6984) (258.1223, 636.2039) (258.0388, 636.8958) (258.0393, 637.7677) (258.2563, 639.8435) (258.448, 642.9686) (258.6792, 647.1359) (258.8204, 651.3077) (258.8923, 655.481) (258.8992, 659.655) (258.8472, 662.4371) (258.8212, 663.8282) knots 0 0 0 0 0.062506 0.125011 0.187517 0.250023 0.312528 0.375034 0.390661 0.406272 0.414085 0.421898 0.429707 0.43752 0.44533 0.453144 0.468748 0.476562 0.484374 0.5 0.515626 0.523438 0.531252 0.546856 0.55467 0.56248 0.570293 0.578102 0.585915 0.593728 0.609339 0.624966 0.687472 0.749977 0.812483 0.874989 0.937494 1 1 1 1 projected
  arc A107 (258.8212, 663.8282) -> (249.3517, 667.4429) centre (0, 0) ccw projected
  spline S104 degree 3 poles (249.3517, 667.4429) (248.4053, 666.423) (246.5127, 664.3832) (243.7365, 661.2662) (241.0092, 658.1066) (238.3347, 654.9019) (235.7302, 651.6405) (233.7907, 649.1825) (232.5693, 647.4901) (231.9887, 646.8396) (231.4654, 646.3793) (231.0302, 646.0904) (230.5786, 645.8271) (230.0921, 645.6356) (229.5936, 645.4793) (228.9073, 645.3585) (228.2058, 645.3582) (227.5178, 645.4682) (226.8518, 645.6733) (226.037, 645.9767) (225.2109, 646.2475) (224.5623, 646.5024) (223.9558, 646.8453) (223.4075, 647.2829) (222.9463, 647.8053) (222.654, 648.2383) (222.393, 648.6914) (222.2041, 649.1788) (222.044, 649.676) (221.9218, 650.3622) (221.8734, 651.2327) (221.9737, 653.3175) (221.9899, 656.4484) (221.9871, 660.6221) (221.8941, 664.7953) (221.7319, 668.966) (221.5048, 673.1339) (221.2968, 675.9087) (221.1928, 677.2961) knots 0 0 0 0 0.062506 0.125011 0.187517 0.250023 0.312528 0.375034 0.390661 0.406272 0.414085 0.421898 0.429707 0.43752 0.44533 0.453144 0.468748 0.476562 0.484374 0.5 0.515626 0.523438 0.531252 0.546856 0.55467 0.56248 0.570293 0.578102 0.585915 0.593728 0.609339 0.624966 0.687472 0.749977 0.812483 0.874989 0.937494 1 1 1 1 projected
  arc A108 (221.1928, 677.2961) -> (211.5356, 680.3741) centre (0, 0) ccw projected
  spline S105 degree 3 poles (211.5356, 680.3741) (210.6479, 679.3028) (208.8726, 677.1601) (206.2756, 673.8923) (203.7298, 670.5848) (201.2391, 667.2351) (198.8216, 663.8328) (197.023, 661.27) (195.8984, 659.5117) (195.3552, 658.8297) (194.8585, 658.3408) (194.4401, 658.028) (194.0041, 657.7397) (193.529, 657.5212) (193.0401, 657.3372) (192.3616, 657.1782) (191.6613, 657.1385) (190.9681, 657.2098) (190.2917, 657.3772) (189.4612, 657.6344) (188.6212, 657.8585) (187.9593, 658.0766) (187.3345, 658.385) (186.7626, 658.7912) (186.2728, 659.2869) (185.9567, 659.7028) (185.6707, 660.1405) (185.4548, 660.6166) (185.267, 661.1041) (185.1066, 661.7823) (185.0095, 662.6487) (184.9927, 664.7358) (184.8333, 667.8628) (184.5965, 672.0298) (184.2697, 676.1911) (183.8738, 680.3462) (183.4134, 684.4948) (183.0502, 687.2536) (182.8686, 688.6329) knots 0 0 0 0 0.062506 0.125011 0.187517 0.250023 0.312528 0.375034 0.390661 0.406272 0.414085 0.421898 0.429707 0.43752 0.44533 0.453144 0.468748 0.476562 0.484374 0.5 0.515626 0.523438 0.531252 0.546856 0.55467 0.56248 0.570293 0.578102 0.585915 0.593728 0.609339 0.624966 0.687472 0.749977 0.812483 0.874989 0.937494 1 1 1 1 projected
  arc A109 (182.8686, 688.6329) -> (173.0539, 691.1647) centre (0, 0) ccw projected
  spline S106 degree 3 poles (173.0539, 691.1647) (172.2277, 690.0452) (170.5754, 687.8064) (168.1656, 684.3981) (165.8093, 680.953) (163.5103, 677.469) (161.2874, 673.9365) (159.6353, 671.2769) (158.6111, 669.4583) (158.1069, 668.7469) (157.6385, 668.2309) (157.2383, 667.8951) (156.8191, 667.5829) (156.357, 667.3381) (155.8792, 667.127) (155.2107, 666.9301) (154.5137, 666.8512) (153.8177, 666.8835) (153.1329, 667.0128) (152.2893, 667.223) (151.438, 667.3996) (150.765, 667.5803) (150.1239, 667.8532) (149.5301, 668.2267) (149.0132, 668.6941) (148.6743, 669.0916) (148.3642, 669.5126) (148.122, 669.9759) (147.9072, 670.452) (147.709, 671.1202) (147.5634, 671.9798) (147.4297, 674.0627) (147.0952, 677.1758) (146.6251, 681.3229) (146.0655, 685.4594) (145.4372, 689.5858) (144.7449, 693.702) (144.2276, 696.4361) (143.9689, 697.8031) knots 0 0 0 0 0.062506 0.125011 0.187517 0.250023 0.312528 0.375034 0.390661 0.406272 0.414085 0.421898 0.429707 0.43752 0.44533 0.453144 0.468748 0.476562 0.484374 0.5 0.515626 0.523438 0.531252 0.546856 0.55467 0.56248 0.570293 0.578102 0.585915 0.593728 0.609339 0.624966 0.687472 0.749977 0.812483 0.874989 0.937494 1 1 1 1 projected
  arc A110 (143.9689, 697.8031) -> (134.0277, 699.7805) centre (0, 0) ccw projected
  spline S107 degree 3 poles (134.0277, 699.7805) (133.2656, 698.6166) (131.7414, 696.2886) (129.5266, 692.7506) (127.3671, 689.1788) (125.2671, 685.5713) (123.2458, 681.9197) (121.7454, 679.1716) (120.8247, 677.2985) (120.3613, 676.56) (119.9225, 676.0185) (119.5418, 675.6608) (119.1407, 675.3255) (118.6931, 675.0552) (118.2279, 674.8177) (117.5715, 674.5836) (116.88, 674.4658) (116.1832, 674.459) (115.4923, 674.5497) (114.6382, 674.7123) (113.7784, 674.8409) (113.0963, 674.9835) (112.4409, 675.22) (111.8271, 675.5596) (111.2848, 675.9973) (110.9241, 676.3752) (110.5909, 676.7782) (110.3231, 677.2271) (110.0819, 677.6905) (109.8466, 678.3465) (109.6531, 679.1966) (109.4027, 681.2687) (108.8942, 684.3582) (108.1923, 688.4724) (107.4016, 692.571) (106.5431, 696.6556) (105.621, 700.7266) (104.9512, 703.4274) (104.6163, 704.7778) knots 0 0 0 0 0.062506 0.125011 0.187517 0.250023 0.312528 0.375034 0.390661 0.406272 0.414085 0.421898 0.429707 0.43752 0.44533 0.453144 0.468748 0.476562 0.484374 0.5 0.515626 0.523438 0.531252 0.546856 0.55467 0.56248 0.570293 0.578102 0.585915 0.593728 0.609339 0.624966 0.687472 0.749977 0.812483 0.874989 0.937494 1 1 1 1 projected
  arc A111 (104.6163, 704.7778) -> (94.5799, 706.1947) centre (0, 0) ccw projected
  spline S108 degree 3 poles (94.5799, 706.1947) (93.8842, 704.9898) (92.4929, 702.58) (90.48, 698.9234) (88.5241, 695.2361) (86.6297, 691.5166) (84.8163, 687.7574) (83.4724, 684.9295) (82.6582, 683.0077) (82.2369, 682.2443) (81.8292, 681.6791) (81.4691, 681.3006) (81.0875, 680.9434) (80.6558, 680.6484) (80.2045, 680.3852) (79.5623, 680.1147) (78.8785, 679.9583) (78.1832, 679.9124) (77.4883, 679.9642) (76.6265, 680.0787) (75.7608, 680.1588) (75.0717, 680.263) (74.4041, 680.4624) (73.7722, 680.7671) (73.2063, 681.1737) (72.825, 681.5307) (72.4697, 681.9144) (72.1771, 682.3476) (71.9103, 682.7967) (71.6386, 683.4385) (71.3977, 684.2764) (71.0316, 686.3312) (70.3506, 689.3873) (69.4192, 693.4557) (68.3999, 697.5035) (67.3136, 701.5336) (66.1648, 705.5465) (65.3446, 708.2054) (64.9345, 709.5349) knots 0 0 0 0 0.062506 0.125011 0.187517 0.250023 0.312528 0.375034 0.390661 0.406272 0.414085 0.421898 0.429707 0.43752 0.44533 0.453144 0.468748 0.476562 0.484374 0.5 0.515626 0.523438 0.531252 0.546856 0.55467 0.56248 0.570293 0.578102 0.585915 0.593728 0.609339 0.624966 0.687472 0.749977 0.812483 0.874989 0.937494 1 1 1 1 projected
  arc A112 (64.9345, 709.5349) -> (54.8344, 710.3868) centre (0, 0) ccw projected
  point P0 (73.8967, 655.85)
  point P1 (-73.8967, 655.85)
  dimension "d7" = 1320
  dimension "d8" = 12.857
  constraints: 6 end point, 2 horizontal alignment, 2 vertical alignment, 1 coincident, 1 vertical, 114 other
  measures "d8" angle of L1 L2
extrude "Extrusion3" cut sketch "Sketch2" against normal through all
sketch "Sketch3" plane through (0, 0, 0) normal (0, 0, 1) x (1, 0, 0)
  circle A0 centre (0, 0) radius 667.5 construction
  line L0 (0, 0) -> (56.1162, 665.137) construction
  line L1 (0, 0) -> (-56.1162, 665.137) construction
  line L2 (0, 0) -> (0, 667.5) construction
  dimension "d11" = 1335
  dimension "d12" = 9.645
  constraints: 6 end point, 3 coincident, 3 point on circle, 1 centre point, 1 vertical, 1 other
  measures "d11" diameter of A0
  measures "d12" angle of L1 L0
hole "Hole1" at (-56.1162, 665.137, 0) at (56.1162, 665.137, 0) direction (0, 0, -1) diameter 8 end through all
equation "\"d7\" = Шстр_диам_внутр"
equation "\"Module\" = 12.5"
equation "\"PressureAngle\" = 20deg"
equation "\"UnitProfileClearance\" = 0.25"
equation "\"UnitRoundRadius\" = 0.35"
equation "\"HeadDiameter\" = 1425"
equation "\"RootDiameter\" = 1368.75"
equation "\"BaseDiameter\" = 1315.56967"
equation "\"HelixAngle\" = 0"
equation "\"UnitCorrection\" = 0"
equation "\"UnitAddendumModification\" = 0"
equation "\"CircularPitch\" = 39.269908"
equation "\"UnitBacklashShift\" = 0"
equation "\"TotalToolShift\" = 0"
equation "\"IsInternal\" = 0"
equation "\"Шстр_диам_внутр\" = 1320"
